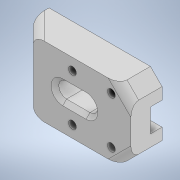
# Autodesk Inventor part: end_tip_2
Saved by Autodesk Inventor 2020 (Build 240168000, 168)
## iProperties
Created: 2019-10-27
Part Number: end_tip_2
Material: Generic
Document SubType Name: Modeling
Designer: psrob
Density: 1 g/cm^3
Appearance: Default
Author: psrob
Autodesk Inventor part; units mm, degrees
ref_plane "YZ Plane" through (0, 0, 0) normal (1, 0, 0) x (0, 1, 0)
ref_plane "XZ Plane" through (0, 0, 0) normal (0, 1, 0) x (-1, 0, 0)
ref_plane "XY Plane" through (0, 0, 0) normal (0, 0, 1) x (1, 0, 0)
sketch "Sketch1" plane through (0, 0, 0) normal (0, 0, 1) x (1, 0, 0)
  line L0 (14.5, -3) -> (-5.5, -3) projected
  line L1 (-5.5, -3) -> (-5.5, 3) projected
  line L2 (-5.5, 3) -> (14.5, 3) projected
  line L3 (14.5, 3) -> (14.5, 9) projected
  line L4 (14.5, 9) -> (-14.5, 9) projected
  line L5 (-14.5, 9) -> (-14.5, 0) projected
  line L6 (-14.5, 0) -> (-14.5, -9) projected
  line L7 (-14.5, -9) -> (14.5, -9) projected
  line L8 (14.5, -9) -> (14.5, -3) projected
  circle A0 centre (-0.5, 6) radius 1 projected
  circle A1 centre (9.5, 6) radius 1 projected
  circle A2 centre (-0.5, -6) radius 1 projected
  circle A3 centre (9.5, -6) radius 1 projected
  point P0 (0, 0)
extrude "Extrusion1" add sketch "Sketch1" along normal blind 3
sketch "Sketch2" plane through (0, 0, 3) normal (0, 0, 1) x (1, 0, 0)
  line L0 (-5.5, -3) -> (-5.5, 3) projected
  line L1 (-5.5, 3) -> (14.5, 3) projected
  line L2 (14.5, 3) -> (14.5, 9) projected
  line L3 (14.5, 9) -> (-14.5, 9) projected
  line L4 (-14.5, 9) -> (-14.5, -9) projected
  line L5 (-14.5, -9) -> (14.5, -9) projected
  line L6 (14.5, -9) -> (14.5, -3) projected
  line L7 (14.5, -3) -> (-5.5, -3) projected
  circle A0 centre (-0.5, 6) radius 1 projected
  circle A1 centre (9.5, 6) radius 1 projected
  circle A2 centre (-0.5, -6) radius 1 projected
  circle A3 centre (9.5, -6) radius 1 projected
  line L8 (14.5, 3) -> (14.5, 9) projected
  line L9 (14.5, -3) -> (14.5, 3)
  point P0 (0, 0)
  constraints: 2 end point, 1 collinear
extrude "Extrusion2" add sketch "Sketch2" along normal blind 5
chamfer "Chamfer1" distance 4 angle 45 1 edges at (-14.5, 0, 8)
fillet "Fillet1" radius 2 2 edges at (-12.5, 9, 6) (-12.5, -9, 6)
chamfer "Chamfer2" distance 3 angle 45 2 edges at (14.5, 9, 4) (14.5, -9, 4)
fillet "Fillet2" radius 2 2 edges at (13, -7.5, 8) (13, 7.5, 8)
sketch "Sketch3" plane through (0, 0, 8) normal (0, 0, 1) x (1, 0, 0)
  line L0 (8.6716, 9) -> (14.5, 3.1716) projected
  line L1 (8.6716, 9) -> (-7.6716, 9) projected
  ellipse E0 centre (-7.6716, 7) end of major axis (-10.5, 7) minor radius 2 (-7.6716, 9) -> (-10.5, 7) ccw projected
  line L2 (-10.5, -7) -> (-10.5, 7) projected
  ellipse E1 centre (-7.6716, -7) end of major axis (-10.5, -7) minor radius 2 (-10.5, -7) -> (-7.6716, -9) ccw projected
  line L3 (-7.6716, -9) -> (8.6716, -9) projected
  line L4 (14.5, -3.1716) -> (8.6716, -9) projected
  line L5 (14.5, -3.1716) -> (14.5, 3.1716) projected
  circle A0 centre (-0.5, 6) radius 1 projected
  circle A1 centre (9.5, 6) radius 1 projected
  circle A2 centre (-0.5, -6) radius 1 projected
  circle A3 centre (9.5, -6) radius 1 projected
  line L6 (-3, 0) -> (3, 0) construction
  line L7 (-3, -2) -> (3, -2)
  line L8 (3, 2) -> (-3, 2)
  arc A4 (-3, 2) -> (-3, -2) centre (-3, 0) ccw
  arc A5 (3, -2) -> (3, 2) centre (3, 0) ccw
  point P0 (0, 0)
  dimension "d12" = 3
  dimension "d13" = 4
  constraints: 8 end point, 4 point on circle, 4 tangent, 2 centre point, 1 horizontal, 1 midpoint, 1 parallel, 2 other
  measures "d12" distance of point (0, 0) L6.end
  measures "d13" diameter of A5
extrude "Extrusion3" cut sketch "Sketch3" against normal blind 5 contours A4 L8 A5 L7
chamfer "Chamfer3" distance 1 angle 45 4 edges at (5, 0, 8) (0, -2, 8) (-5, 0, 8) (0, 2, 8)
body "Solid1"
